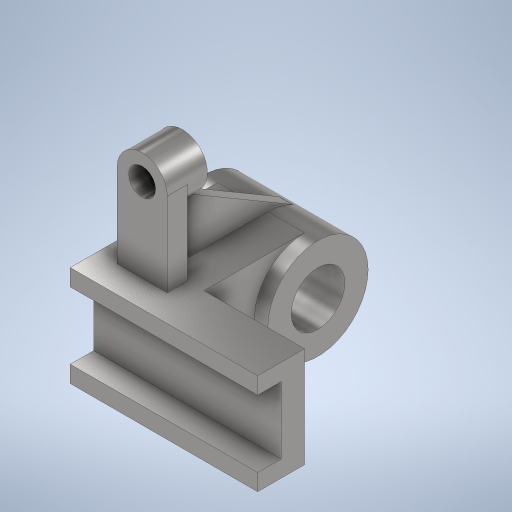
# Autodesk Inventor part: Gary
Saved by Autodesk Inventor 2024 (Build 280153000, 153)
## iProperties
Created: 2024-02-01
Part Number: Gary
Material: Stahl, galvanisiert
Document SubType Name: Modeling
Designer: ffogue
Density: 7.85 g/cm^3
Appearance: Galvanisiert
Author: ffogue
Autodesk Inventor part; units mm, degrees
sketch "Skizze1" plane through (0, 0, 0) normal (0, 0, 1) x (1, 0, 0)
  line L0 (0, 0) -> (112, 0)
  line L1 (112, 0) -> (112, 28)
  line L2 (112, 28) -> (0, 28)
  line L3 (0, 28) -> (0, 0)
  dimension "d0" = 28
  dimension "d1" = 112
  constraints: 8 end point, 2 parallel, 1 horizontal, 1 perpendicular
  measures "d0" distance between parallel lines of L0 L2
  measures "d1" distance between parallel lines of L1 L3
extrude "Extrusion1" add sketch "Skizze1" along normal blind 60
sketch "Skizze2" plane through (112, 0, 0) normal (1, 0, 0) x (0, 0, -1)
  line L0 (0, 0) -> (-60, 0) projected
  line L1 (-50, 0) -> (-50, 14)
  line L2 (-50, 14) -> (-10, 14)
  line L3 (-10, 14) -> (-10, 0)
  line L4 (-60, 0) -> (-60, 28) projected
  line L5 (0, 28) -> (-60, 28) projected
  point P0 (-10, 7)
  point P1 (-50, 7)
  point P2 (-30, 14)
  dimension "d4" = 40
  dimension "d5" = 10
  dimension "d6" = 14
  constraints: 6 end point, 3 midpoint, 2 perpendicular, 2 point on line, 1 vertical
  measures "d4" distance from line of point (-10, 7) L1
  measures "d5" distance from line of point (-50, 7) L4
  measures "d6" distance from line of L5 point (-30, 14)
extrude "Extrusion2" cut sketch "Skizze2" against normal up to surface (112 mm away)
sketch "Skizze3" plane through (0, 28, 0) normal (0, 1, 0) x (1, 0, 0)
  line L0 (112, -60) -> (0, -60) projected
  line L1 (0, 0) -> (112, 0) projected
  line L2 (0, -60) -> (52, -60)
  line L3 (52, -60) -> (52, 0)
  line L4 (52, 0) -> (0, 0)
  line L5 (0, 0) -> (0, -60)
  line L6 (112, 0) -> (112, -60) projected
  point P0 (52, -30)
  dimension "d9" = 60
  constraints: 8 end point, 2 parallel, 1 horizontal, 1 midpoint, 1 perpendicular, 1 point on line
  measures "d9" distance from line of L6 point (52, -30)
extrude "Extrusion3" add sketch "Skizze3" along normal blind 60 contours L0 L5 L1 L3
ref_plane "Arbeitsebene1" through (60, 0, 0) normal (1, 0, 0) x (0, 1, 0)
sketch "Skizze7" plane through (60, 0, 0) normal (1, 0, 0) x (0, 1, 0)
  circle A0 centre (88, 30) radius 30
  circle A1 centre (88, 30) radius 16
  line L0 (28, 0) -> (28, 60) projected
  point P0 (0, 0)
  point P1 (28, 30)
  point P2 (28, 30)
  dimension "d25" = 60
  dimension "d26" = 32
  dimension "d27" = 60
  constraints: 2 centre point, 2 midpoint, 1 coincident, 1 horizontal alignment
  measures "d25" diameter of A0
  measures "d26" diameter of A1
  measures "d27" distance of point (28, 30) A0.centre
extrude "Extrusion6" add sketch "Skizze7" against normal blind 68
extrude "Extrusion7" cut sketch "Skizze7" against normal blind 68 contours A1
ref_plane "Arbeitsebene2" through (0, 16, 0) normal (0, 1, 0) x (-1, 0, 0)
sketch "Skizze11" plane through (0, 16, 0) normal (0, 1, 0) x (-1, 0, 0)
  circle A0 centre (-27, 110) radius 15
  circle A1 centre (-27, 110) radius 8
  line L0 (-12, 110) -> (-12, 59.6136)
  line L1 (-42, 110) -> (-42, 59.6136)
  line L2 (-52, 60) -> (-52, 14) projected
  line L3 (0, 60) -> (-52, 60) projected
  point P0 (0, 0)
  point P1 (-52, 54)
  point P2 (-42, 60)
  point P3 (-12, 60)
  dimension "d42" = 30
  dimension "d43" = 16
  dimension "d44" = 10
  dimension "d45" = 50
  constraints: 4 end point, 2 centre point, 2 point on circle, 2 tangent, 2 vertical, 1 coincident, 1 parallel
  measures "d42" diameter of A0
  measures "d43" diameter of A1
  measures "d44" distance between parallel lines of L2 L1
  measures "d45" distance from line of L3 A0.centre
extrude "Extrusion10" add sketch "Skizze11" along normal blind 24 contours A0
extrude "Extrusion11" add sketch "Skizze11" along normal blind 12 contours L0 L3 L1 A0
ref_plane "Arbeitsebene3" through (30, 0, 0) normal (1, 0, 0) x (0, 1, 0)
sketch "Skizze13" plane through (30, 0, 0) normal (1, 0, 0) x (0, 1, 0)
  line L0 (28, 95) -> (28, 110) projected
  line L1 (31, 56.123) -> (103, 56.123)
  line L2 (103, 56.123) -> (37, 95)
  line L3 (37, 95) -> (28, 95)
  line L4 (28, 95) -> (28, 56.123)
  line L5 (31, 56.123) -> (28, 56.123)
  line L6 (16, 110) -> (28, 110) projected
  line L7 (16, 110) -> (16, 110) projected
  line L8 (16, 110) -> (28, 110) projected
  line L9 (28, 110) -> (28, 110) projected
  line L10 (40, 95) -> (40, 125) projected
  line L11 (28, 95) -> (40, 95) projected
  point P0 (0, 0)
  point P1 (34, 95)
  dimension "d55" = 30.5
  dimension "d56" = 66
  dimension "d57" = 72
  dimension "d58" = 3
  constraints: 10 end point, 2 perpendicular, 2 point on line, 1 midpoint, 1 parallel, 1 vertical
  measures "d55" angle of L1 L2
  measures "d56" horizontal distance of L2.end L1.end
  measures "d57" distance of L1.start L1.end
  measures "d58" distance from line of L2.end L10
extrude "Extrusion12" add sketch "Skizze13" against normal blind 8
